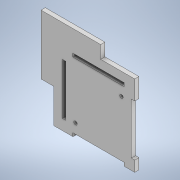
# Autodesk Inventor part: holder4hakon
Saved by Autodesk Inventor 2022.1 (Build 261234000, 234)
## iProperties
Created: 2021-11-10
Part Number: holder4hakon
Material: Generic
Document SubType Name: Modeling
Designer: stein
Density: 1 g/cm^3
Appearance: Default
Author: stein
Autodesk Inventor part; units mm, degrees
ref_plane "YZ Plane" through (0, 0, 0) normal (1, 0, 0) x (0, 1, 0)
ref_plane "XZ Plane" through (0, 0, 0) normal (0, 1, 0) x (-1, 0, 0)
ref_plane "XY Plane" through (0, 0, 0) normal (0, 0, 1) x (1, 0, 0)
sketch "Sketch1" plane through (0, 0, 0) normal (0, 0, 1) x (1, 0, 0)
  line L0 (0, 0) -> (85, 0)
  line L1 (85, 0) -> (85, 85)
  line L2 (85, 85) -> (0, 85)
  line L3 (0, 85) -> (0, 0)
  line L4 (12.5, 85) -> (72.5, 85)
  line L5 (72.5, 85) -> (72.5, 81)
  line L6 (72.5, 81) -> (12.5, 81)
  line L7 (12.5, 81) -> (12.5, 85)
  line L8 (42.5, 0) -> (42.5, 85) construction
  line L9 (0, 42.5) -> (85, 42.5) construction
  line L10 (0, 85) -> (85, 85)
  line L11 (72.5, 0) -> (72.5, 4)
  line L12 (72.5, 4) -> (12.5, 4)
  line L13 (12.5, 4) -> (12.5, 0)
  line L14 (0, 72.5) -> (4, 72.5)
  line L15 (4, 72.5) -> (4, 12.5)
  line L16 (4, 12.5) -> (0, 12.5)
  line L17 (0, 12.5) -> (0, 72.5)
  line L18 (85, 72.5) -> (81, 72.5)
  line L19 (81, 72.5) -> (81, 12.5)
  line L20 (81, 12.5) -> (85, 12.5)
  line L21 (0, 0) -> (-10, 0)
  line L22 (-10, 0) -> (-10, 40)
  line L23 (-10, 40) -> (0, 40)
  line L24 (0, 40) -> (0, 0)
  line L25 (0, 40) -> (-25, 40)
  line L26 (-25, 40) -> (-25, 110)
  line L27 (-25, 110) -> (0, 110)
  line L28 (0, 110) -> (0, 40)
  line L29 (0, 110) -> (45, 110)
  line L30 (45, 110) -> (45, 85)
  line L31 (45, 85) -> (0, 85)
  line L32 (0, 85) -> (0, 110)
  line L33 (85, 85) -> (45, 85)
  line L34 (45, 85) -> (45, 95)
  line L35 (45, 95) -> (85, 95)
  line L36 (85, 95) -> (85, 85)
  point P0 (2, 12.5)
  point P1 (0, 12.5)
  dimension "d0" = 85
  dimension "d1" = 85
  dimension "d2" = 60
  dimension "d3" = 4
  dimension "d4" = 12.5
  dimension "d5" = 4
  dimension "d6" = 60
  dimension "d7" = 12.5
  dimension "d8" = 10
  dimension "d9" = 40
  dimension "d10" = 25
  dimension "d11" = 25
  dimension "d12" = 40
  dimension "d13" = 10
  constraints: 74 end point, 14 parallel, 8 symmetric about line, 7 horizontal, 7 perpendicular, 5 midpoint, 4 point on line
  measures "d0" distance of L2.end L1.end
  measures "d1" distance of L1.end L0.end
  measures "d2" distance of L5.end L6.end
  measures "d3" distance of L4.end L5.end
  measures "d4" distance from line of L3 L6.end
  measures "d5" distance of L15.end L16.end
  measures "d6" distance of L14.end L15.end
  measures "d7" distance from line of L0 point (2, 12.5)
  measures "d8" distance of L22.end L23.end
  measures "d9" distance of L21.end L22.end
  measures "d10" distance of L26.end L27.end
  measures "d11" distance between parallel lines of L27 L2
  measures "d12" distance of L34.end L35.end
  measures "d13" distance of L33.end L34.end
extrude "Extrusion1" add sketch "Sketch1" along normal blind 5 contours L3 L16 L15 L14 L2 L7 L6 L5 L1 L18 L19 L20 L0 L11 L12 L13 | L21 L22 L23 L3 | L23 L25 L26 L27 L28 L3 | L28 L29 L30 L2 | L2 L30 L35 L36
sketch "Sketch2" plane through (0, 0, 5) normal (0, 0, 1) x (1, 0, 0)
  circle A0 centre (15.5, 15.5) radius 2
  circle A1 centre (69.5, 69.5) radius 2
  line L0 (85, 72.5) -> (85, 95) projected
  line L1 (12.5, 85) -> (72.5, 85) projected
  line L2 (12.5, 4) -> (72.5, 4) projected
  line L3 (0, 12.5) -> (0, 72.5) projected
  point P0 (0, 0)
  dimension "d16" = 4
  dimension "d17" = 4
  dimension "d18" = 15.5
  dimension "d19" = 15.5
  dimension "d20" = 11.5
  dimension "d21" = 15.5
  constraints: 2 centre point
  measures "d16" diameter of A0
  measures "d17" diameter of A1
  measures "d18" distance from line of L0 A1.centre
  measures "d19" distance from line of L1 A1.centre
  measures "d20" distance from line of L2 A0.centre
  measures "d21" distance from line of L3 A0.centre
extrude "Extrusion2" cut sketch "Sketch2" against normal through all
body "Solid1"
